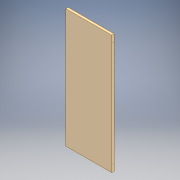
# Autodesk Inventor part: InsulatorWallNorrowasa
Saved by Autodesk Inventor 2017 (Build 210142000, 142)
## iProperties
Created: 2016-12-13
Part Number: InsulatorWallNorrowasa
Material: Polyethylene, Low Density
Document SubType Name: Modeling
Designer: umr
Density: 0.894 g/cm^3
Appearance: Smooth - Off-White
Author: umr
Autodesk Inventor part; units mm, degrees
ref_plane "YZ Plane" through (0, 0, 0) normal (1, 0, 0) x (0, 1, 0)
sketch "Sketch1" plane through (0, 0, 0) normal (0, 1, 0) x (-1, 0, 0)
  line L0 (0, 0) -> (1000, 0)
  line L1 (1000, 0) -> (1000, -2600)
  line L2 (1000, -2600) -> (0, -2600)
  line L3 (0, -2600) -> (0, 0)
  dimension "d0" = 1000
  dimension "d1" = 2600
  constraints: 8 end point, 2 parallel, 1 horizontal, 1 perpendicular
  measures "d0" distance of L1.end L2.end
  measures "d1" distance of L0.end L1.end
extrude "Extrusion1" add sketch "Sketch1" along normal blind 50
sketch "Sketch2" plane through (0, 0, 0) normal (1, 0, 0) x (0, 0, -1)
  circle A0 centre (150, 25) radius 4.25
  line L0 (2600, 0) -> (0, 0) projected
  line L1 (0, 0) -> (0, 50) projected
  dimension "d4" = 8.5
  dimension "d5" = 25
  dimension "d8" = 150
  constraints: 1 centre point
  measures "d4" diameter of A0
  measures "d5" distance from line of L0 A0.centre
  measures "d8" distance from line of L1 A0.centre
extrude "Extrusion2" cut sketch "Sketch2" against normal blind 10
ref_plane "Work Plane2" through (-1000, 0, -1300) normal (0, 0, 1) x (1, 0, 0)
ref_plane "Work Plane3" through (-500, 0, -2600) normal (-1, 0, 0) x (0, 0, 1)
mirror "Mirror1" about plane through (-1000, 0, -1300) normal (0, 0, 1) of "Extrusion2"
mirror "Mirror2" about plane through (-500, 0, -2600) normal (-1, 0, 0) of "Extrusion2", "Mirror1"
body "Solid1"
